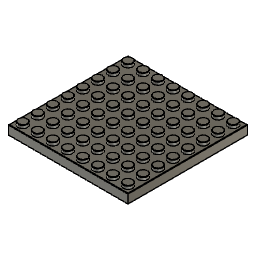
8x8block (Autodesk Fusion 360 design; units mm, degrees)
Autodesk Fusion 360 part; units mm, degrees
sketch "Sketch1" plane through (0, 0, 0) normal (0, 0, 1) x (1, 0, 0)
  line L0 (0, 0) -> (63.8, 0)
  line L1 (63.8, 0) -> (63.8, 63.8)
  line L2 (63.8, 63.8) -> (0, 63.8)
  line L3 (0, 63.8) -> (0, 0)
  constraint coincident L0.start L3.end
extrude "Extrude1" add sketch "Sketch1" along normal blind 4.8
sketch "Sketch2" plane through (0, 0, 4.8) normal (0, 0, 1) x (-1, 0, 0)
  line L0 (0, -63.8) -> (0, 0)
  line L1 (0, 0) -> (-63.8, 0)
  line L2 (-63.8, 0) -> (-63.8, -63.8)
  line L3 (-63.8, -63.8) -> (0, -63.8)
  circle A0 centre (-3.9, -59.9) radius 2.5
extrude "Extrude2" add sketch "Sketch2" along normal blind 1.7 contours A0
fillet "Fillet1" radius 0.2 1 edges at (6.2308, 60.804, 6.5)
pattern_linear "R-Pattern1" count 8 spacing 8.0286 along (1, 0, 0) count 8 spacing 8.0286 along (0, -1, 0) of "Extrude2"
shell "Shell1" thickness 1.49 removed faces 1 at (21.2667, 21.2667, 0)
sketch "Sketch3" plane through (0, 0, 3.31) normal (0, 0, -1) x (1, 0, 0)
  circle A0 centre (60.1, -3.7) radius 1.01
  circle A1 centre (52.0714, -3.7) radius 1.01
  circle A2 centre (44.0429, -3.7) radius 1.01
  circle A3 centre (36.0143, -3.7) radius 1.01
  circle A4 centre (27.9857, -3.7) radius 1.01
  circle A5 centre (19.9571, -3.7) radius 1.01
  circle A6 centre (11.9286, -3.7) radius 1.01
  circle A7 centre (3.9, -3.7) radius 1.01
  circle A8 centre (60.1, -11.7286) radius 1.01
  circle A9 centre (52.0714, -11.7286) radius 1.01
  circle A10 centre (44.0429, -11.7286) radius 1.01
  circle A11 centre (36.0143, -11.7286) radius 1.01
  circle A12 centre (27.9857, -11.7286) radius 1.01
  circle A13 centre (19.9571, -11.7286) radius 1.01
  circle A14 centre (11.9286, -11.7286) radius 1.01
  circle A15 centre (3.9, -11.7286) radius 1.01
  circle A16 centre (60.1, -19.7571) radius 1.01
  circle A17 centre (52.0714, -19.7571) radius 1.01
  circle A18 centre (44.0429, -19.7571) radius 1.01
  circle A19 centre (36.0143, -19.7571) radius 1.01
  circle A20 centre (27.9857, -19.7571) radius 1.01
  circle A21 centre (19.9571, -19.7571) radius 1.01
  circle A22 centre (11.9286, -19.7571) radius 1.01
  circle A23 centre (3.9, -19.7571) radius 1.01
  circle A24 centre (60.1, -27.7857) radius 1.01
  circle A25 centre (52.0714, -27.7857) radius 1.01
  circle A26 centre (44.0429, -27.7857) radius 1.01
  circle A27 centre (36.0143, -27.7857) radius 1.01
  circle A28 centre (27.9857, -27.7857) radius 1.01
  circle A29 centre (19.9571, -27.7857) radius 1.01
  circle A30 centre (11.9286, -27.7857) radius 1.01
  circle A31 centre (3.9, -27.7857) radius 1.01
  circle A32 centre (60.1, -35.8143) radius 1.01
  circle A33 centre (52.0714, -35.8143) radius 1.01
  circle A34 centre (44.0429, -35.8143) radius 1.01
  circle A35 centre (36.0143, -35.8143) radius 1.01
  circle A36 centre (27.9857, -35.8143) radius 1.01
  circle A37 centre (19.9571, -35.8143) radius 1.01
  circle A38 centre (11.9286, -35.8143) radius 1.01
  circle A39 centre (3.9, -35.8143) radius 1.01
  circle A40 centre (60.1, -43.8429) radius 1.01
  circle A41 centre (52.0714, -43.8429) radius 1.01
  circle A42 centre (44.0429, -43.8429) radius 1.01
  circle A43 centre (36.0143, -43.8429) radius 1.01
  circle A44 centre (27.9857, -43.8429) radius 1.01
  circle A45 centre (19.9571, -43.8429) radius 1.01
  circle A46 centre (11.9286, -43.8429) radius 1.01
  circle A47 centre (3.9, -43.8429) radius 1.01
  circle A48 centre (60.1, -51.8714) radius 1.01
  circle A49 centre (52.0714, -51.8714) radius 1.01
  circle A50 centre (44.0429, -51.8714) radius 1.01
  circle A51 centre (36.0143, -51.8714) radius 1.01
  circle A52 centre (27.9857, -51.8714) radius 1.01
  circle A53 centre (19.9571, -51.8714) radius 1.01
  circle A54 centre (11.9286, -51.8714) radius 1.01
  circle A55 centre (3.9, -51.8714) radius 1.01
  circle A56 centre (60.1, -59.9) radius 1.01
  circle A57 centre (52.0714, -59.9) radius 1.01
  circle A58 centre (44.0429, -59.9) radius 1.01
  circle A59 centre (36.0143, -59.9) radius 1.01
  circle A60 centre (27.9857, -59.9) radius 1.01
  circle A61 centre (19.9571, -59.9) radius 1.01
  circle A62 centre (11.9286, -59.9) radius 1.01
  circle A63 centre (3.9, -59.9) radius 1.01
  line L0 (1.49, -1.49) -> (1.49, -62.31)
  line L1 (1.49, -62.31) -> (62.31, -62.31)
  line L2 (62.31, -62.31) -> (62.31, -1.49)
  line L3 (62.31, -1.49) -> (1.49, -1.49)
  circle A64 centre (7.9143, -7.7143) radius 3.15
  circle A65 centre (7.9143, -7.7143) radius 2.15
extrude "Extrude3" add sketch "Sketch3" along normal blind 3.3 contours A64
pattern_linear "R-Pattern2" count 7 spacing 8.0333 along (1, 0, 0) count 7 spacing 8.0333 along (0, 1, 0) of "Extrude3"
fillet "Fillet2" radius 0.2 67 edges at (31.9, 63.8, 4.8) (0, 31.9, 4.8) (31.9, 0, 4.8) (63.8, 31.9, 4.8) (62.4308, 4.604, 6.5) (62.4308, 12.6326, 6.5) (62.4308, 20.6612, 6.5) (62.4308, 28.6898, 6.5) (62.4308, 36.7183, 6.5) (62.4308, 44.7469, 6.5) (62.4308, 52.7755, 6.5) (62.4308, 60.804, 6.5) (54.4022, 60.804, 6.5) (54.4022, 52.7755, 6.5) (54.4022, 44.7469, 6.5) (54.4022, 36.7183, 6.5) (54.4022, 28.6898, 6.5) (54.4022, 20.6612, 6.5) (54.4022, 12.6326, 6.5) (54.4022, 4.604, 6.5) (46.3737, 4.604, 6.5) (46.3737, 12.6326, 6.5) (46.3737, 20.6612, 6.5) (46.3737, 28.6898, 6.5) (46.3737, 36.7183, 6.5) (46.3737, 44.7469, 6.5) (46.3737, 52.7755, 6.5) (46.3737, 60.804, 6.5) (38.3451, 60.804, 6.5) (38.3451, 52.7755, 6.5) (38.3451, 44.7469, 6.5) (38.3451, 36.7183, 6.5) (38.3451, 28.6898, 6.5) (38.3451, 20.6612, 6.5) (38.3451, 12.6326, 6.5) (38.3451, 4.604, 6.5) (30.3165, 4.604, 6.5) (30.3165, 12.6326, 6.5) (30.3165, 20.6612, 6.5) (30.3165, 28.6898, 6.5) (30.3165, 36.7183, 6.5) (30.3165, 44.7469, 6.5) (30.3165, 52.7755, 6.5) (30.3165, 60.804, 6.5) (22.288, 60.804, 6.5) (22.288, 52.7755, 6.5) (22.288, 44.7469, 6.5) (22.288, 36.7183, 6.5) (22.288, 28.6898, 6.5) (22.288, 20.6612, 6.5) (22.288, 12.6326, 6.5) (22.288, 4.604, 6.5) (14.2594, 4.604, 6.5) (14.2594, 12.6326, 6.5) (14.2594, 20.6612, 6.5) (14.2594, 28.6898, 6.5) (14.2594, 36.7183, 6.5) (14.2594, 44.7469, 6.5) (14.2594, 52.7755, 6.5) (14.2594, 60.804, 6.5) (6.2308, 52.7755, 6.5) (6.2308, 44.7469, 6.5) (6.2308, 36.7183, 6.5) (6.2308, 28.6898, 6.5) (6.2308, 20.6612, 6.5) (6.2308, 12.6326, 6.5) (6.2308, 4.604, 6.5)
scale "Scale1" factor 0.75 about (29.8643, 31.8143, 3.31) bodies 1
